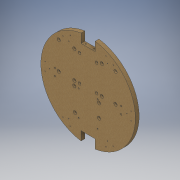
# Autodesk Inventor part: Platte3_neu
Saved by Autodesk Inventor 2017 SP1 (Build 210196100, 196)
## iProperties
Part Number: Platte3_neu
Material: Generisch
Document SubType Name: Modeling
Designer: Alex
Density: 1 g/cm^3
Appearance: Holzplatte
Author: Alex
Autodesk Inventor part; units mm, degrees
ref_plane "YZ Plane" through (0, 0, 0) normal (1, 0, 0) x (0, 1, 0)
ref_plane "XZ Plane" through (0, 0, 0) normal (0, 1, 0) x (-1, 0, 0)
ref_plane "XY Plane" through (0, 0, 0) normal (0, 0, 1) x (1, 0, 0)
sketch "Skizze1" plane through (0, 0, 0) normal (0, 1, 0) x (-1, 0, 0)
  circle A0 centre (0, 0) radius 100
  dimension "d0" = 200
  constraints: 1 centre point, 1 coincident
  measures "d0" diameter of A0
extrude "Extrusion1" add sketch "Skizze1" along normal blind 8
sketch "Skizze3" plane through (0, 0, 0) normal (0, -1, 0) x (1, 0, 0)
  point P0 (0, 0)
  point P1 (91, 8.85)
  point P2 (91, -8.85)
  point P3 (82, 0)
  point P4 (37.8357, 83.2333)
  point P5 (41, 71.0141)
  point P6 (53.1643, 74.3833)
  point P7 (-53.1643, 74.3833)
  point P8 (-41, 71.0141)
  point P9 (-37.8357, 83.2333)
  point P10 (-91, -8.85)
  point P11 (-82, 0)
  point P12 (-91, 8.85)
  point P13 (-37.8357, -83.2333)
  point P14 (-41, -71.0141)
  point P15 (-53.1643, -74.3833)
  point P16 (53.1643, -74.3833)
  point P17 (41, -71.0141)
  point P18 (37.8357, -83.2333)
  dimension "d3" = 17.7
  dimension "d4" = 9
  dimension "d5" = 8.85
  dimension "d6" = 82
  dimension "d9" = 360
  constraints: 1 horizontal alignment, 1 vertical alignment, 19 other
  measures "d3" distance of point (91, -8.85) point (91, 8.85)
  measures "d4" horizontal distance of point (82, 0) point (91, 8.85)
  measures "d5" vertical distance of point (82, 0) point (91, 8.85)
  measures "d6" distance of point (0, 0) point (82, 0)
hole "Bohrung1" at (91, 0, 8.85) at (91, 0, -8.85) at (82, 0, 0) at (37.8357, 0, 83.2333) at (41, 0, 71.0141) at (53.1643, 0, 74.3833) at (-53.1643, 0, 74.3833) at (-41, 0, 71.0141) at (-37.8357, 0, 83.2333) at (-91, 0, -8.85) at (-82, 0, 0) at (-91, 0, 8.85) at (-37.8357, 0, -83.2333) at (-41, 0, -71.0141) at (-53.1643, 0, -74.3833) at (53.1643, 0, -74.3833) at (41, 0, -71.0141) at (37.8357, 0, -83.2333) direction (0, 1, 0) diameter 1.5 depth 5 tip angle 118
sketch "Skizze4" plane through (0, 0, 0) normal (0, -1, 0) x (1, 0, 0)
  line L0 (0, 140.1034) -> (0, 25.1034)
  line L1 (0, 80) -> (15, 80)
  line L2 (15, 80) -> (15, 98.8686)
  circle A0 centre (0, 0) radius 100 projected
  arc A1 (15, 98.8686) -> (0, 100) centre (0, 0) ccw
  line L3 (0, 80) -> (-15, 80)
  line L4 (-15, 80) -> (-15, 98.8686)
  arc A2 (0, 100) -> (-15, 98.8686) centre (0, 0) ccw
  line L5 (0, -80) -> (-15, -80)
  line L6 (-15, -80) -> (-15, -98.8686)
  line L7 (0, -80) -> (15, -80)
  line L8 (15, -80) -> (15, -98.8686)
  arc A3 (-15, -98.8686) -> (0, -100) centre (0, 0) ccw
  arc A4 (0, -100) -> (15, -98.8686) centre (0, 0) ccw
  dimension "d18" = 15
  dimension "d20" = 80
  dimension "d27" = 15
  dimension "d28" = 15
  constraints: 18 end point, 8 point on circle, 4 centre point, 3 symmetric about line, 2 point on line, 1 coincident, 1 horizontal, 1 perpendicular, 1 vertical, 1 vertical alignment, 3 other
  measures "d18" distance of L1.start L1.end
  measures "d20" distance from line of point (0, 0) L1
  measures "d27" distance of L5.start L7.end
  measures "d28" distance of L5.start L5.end
extrude "Extrusion2" cut sketch "Skizze4" against normal blind 8 contours A0 L2 L1 L0 | L0 L3 L4 A0 | L6 L5 L7 L8 A0
sketch "Skizze5" plane through (-15, 0, 80) normal (0, 0, 1) x (1, 0, 0)
  line L0 (30, 8) -> (30, 0) projected
  line L1 (0, 8) -> (30, 8) projected
  point P0 (15, 0)
  point P1 (23.75, 4)
  point P2 (6.25, 4)
  dimension "d29" = 17.5
  dimension "d30" = 6.25
  dimension "d31" = 4
  constraints: 1 horizontal alignment
  measures "d29" distance of point (6.25, 4) point (23.75, 4)
  measures "d30" distance from line of point (23.75, 4) L0
  measures "d31" distance from line of L1 point (23.75, 4)
sketch "Skizze6" plane through (15, 0, -80) normal (0, 0, -1) x (-1, 0, 0)
  point P0 (15, 0)
  point P1 (6.25, 4)
  point P2 (23.75, 4)
hole "Bohrung2" at (8.75, 4, -80) at (-8.75, 4, -80) direction (0, 0, 1) diameter 2 depth 10 tip angle 118
hole "Bohrung3" at (8.75, 4, 80) at (-8.75, 4, 80) direction (0, 0, -1) diameter 2 depth 10 tip angle 118
sketch "Skizze11" plane through (0, 0, 0) normal (0, -1, 0) x (1, 0, 0)
  point P0 (0, 0)
  point P1 (20, -5)
  point P2 (-20, -5)
  point P3 (20, -59)
  point P4 (-20, -59)
  dimension "d81" = 40
  dimension "d82" = 20
  dimension "d83" = 5
  dimension "d84" = 54
  constraints: 2 horizontal alignment, 2 vertical alignment
  measures "d81" distance of point (-20, -5) point (20, -5)
  measures "d82" horizontal distance of point (0, 0) point (-20, -5)
  measures "d83" vertical distance of point (0, 0) point (-20, -5)
  measures "d84" distance of point (-20, -59) point (-20, -5)
hole "Bohrung5" at (20, 0, -5) at (-20, 0, -5) at (20, 0, -59) at (-20, 0, -59) direction (0, 1, 0) diameter 2.5 depth 8 tip angle 118
chamfer "Fase1" distance 2 angle 45 4 edges at (20, 8, -3.75) (-20, 8, -3.75) (-20, 8, -57.75) (20, 8, -57.75)
sketch "Skizze13" plane through (0, 0, 0) normal (0, -1, 0) x (1, 0, 0)
  point P0 (0, 0)
  point P1 (70, -7.5)
  point P2 (70, 7.5)
  point P3 (-70, -7.5)
  point P4 (-70, 7.5)
  dimension "d95" = 15
  dimension "d96" = 7.5
  dimension "d97" = 70
  dimension "d100" = 360
  constraints: 1 vertical alignment, 5 other
  measures "d95" distance of point (70, 7.5) point (70, -7.5)
  measures "d96" vertical distance of point (0, 0) point (70, -7.5)
  measures "d97" horizontal distance of point (0, 0) point (70, -7.5)
hole "Bohrung6" at (70, 0, -7.5) at (70, 0, 7.5) at (-70, 0, -7.5) at (-70, 0, 7.5) direction (0, 1, 0) diameter 3 depth 8 tip angle 118
chamfer "Fase2" distance 2 angle 45 4 edges at (70, 8, 9) (70, 8, -6) (-70, 8, -6) (-70, 8, 9)
sketch "Skizze14" plane through (0, 0, 0) normal (0, -1, 0) x (1, 0, 0)
  point P0 (0, 0)
  point P1 (29, -54)
  point P2 (29, -5)
  point P3 (-29, -5)
  point P4 (-29, -54)
  dimension "d112" = 49
  dimension "d113" = 58
  dimension "d114" = 5
  dimension "d115" = 29
  constraints: 2 horizontal alignment, 2 vertical alignment
  measures "d112" distance of point (-29, -5) point (-29, -54)
  measures "d113" distance of point (-29, -54) point (29, -54)
  measures "d114" vertical distance of point (0, 0) point (-29, -5)
  measures "d115" horizontal distance of point (0, 0) point (-29, -5)
hole "Bohrung7" [suppressed]
chamfer "Fase3" [suppressed]
sketch "Skizze15" plane through (0, 0, 0) normal (0, -1, 0) x (1, 0, 0)
  point P0 (0, 0)
  point P1 (58, 5)
  point P2 (58, 65)
  point P3 (29, 65)
  point P4 (29, 5)
  dimension "d126" = 29
  dimension "d127" = 60
  dimension "d128" = 5
  dimension "d129" = 29
  constraints: 2 horizontal alignment, 2 vertical alignment
  measures "d126" distance of point (29, 5) point (58, 5)
  measures "d127" distance of point (29, 65) point (29, 5)
  measures "d128" vertical distance of point (0, 0) point (29, 5)
  measures "d129" horizontal distance of point (0, 0) point (29, 5)
hole "Bohrung8" at (58, 0, 5) at (58, 0, 65) at (29, 0, 65) at (29, 0, 5) direction (0, 1, 0) diameter 3 depth 8 tip angle 118
chamfer "Fase4" distance 2 angle 45 4 edges at (29, 0, 6.5) (58, 0, 6.5) (58, 0, 66.5) (29, 0, 66.5)
sketch "Skizze16" plane through (0, 0, 0) normal (0, -1, 0) x (1, 0, 0)
  point P0 (0, 0)
  point P1 (-29, 5)
  point P2 (-29, 63)
  point P3 (-62, 63)
  point P4 (-62, 5)
  dimension "d140" = 33
  dimension "d141" = 58
  dimension "d142" = 5
  dimension "d143" = 29
  constraints: 2 horizontal alignment, 2 vertical alignment
  measures "d140" distance of point (-62, 5) point (-29, 5)
  measures "d141" distance of point (-29, 63) point (-29, 5)
  measures "d142" vertical distance of point (0, 0) point (-29, 5)
  measures "d143" horizontal distance of point (0, 0) point (-29, 5)
hole "Bohrung9" at (-29, 0, 5) at (-29, 0, 63) at (-62, 0, 63) at (-62, 0, 5) direction (0, 1, 0) diameter 3 depth 8 tip angle 118
chamfer "Fase5" distance 2 angle 45 4 edges at (-62, 0, 6.5) (-29, 0, 6.5) (-29, 0, 64.5) (-62, 0, 64.5)
sketch "Skizze17" plane through (0, 0, 0) normal (0, -1, 0) x (1, 0, 0)
  point P0 (0, 0)
  point P1 (-18, 5)
  point P2 (18, 5)
  point P3 (18, 61)
  point P4 (-18, 61)
  dimension "d154" = 56
  dimension "d155" = 36
  dimension "d156" = 18
  dimension "d157" = 5
  constraints: 2 horizontal alignment, 2 vertical alignment
  measures "d154" distance of point (-18, 61) point (-18, 5)
  measures "d155" distance of point (-18, 5) point (18, 5)
  measures "d156" horizontal distance of point (0, 0) point (-18, 5)
  measures "d157" vertical distance of point (0, 0) point (-18, 5)
hole "Bohrung10" at (-18, 0, 5) at (18, 0, 5) at (18, 0, 61) at (-18, 0, 61) direction (0, 1, 0) diameter 2 depth 8 tip angle 118
chamfer "Fase6" distance 2 angle 45 4 edges at (-18, 0, 6) (-18, 0, 62) (18, 0, 62) (18, 0, 6)
sketch "Skizze19" plane through (0, 0, 0) normal (0, -1, 0) x (1, 0, 0)
  circle A0 centre (-29, -5) radius 1.5 projected
  point P0 (0, 0)
  point P1 (-27.73, -53.277)
  point P2 (23.07, -38.02)
  point P3 (23.07, -10.08)
  dimension "d168" = 48.277
  dimension "d170" = 27.94
  dimension "d172" = 5.08
  dimension "d186" = 1.27
  dimension "d187" = 52.07
  constraints: 1 coincident, 1 vertical alignment
  measures "d168" vertical distance of point (-29, -5) point (-27.73, -53.277)
  measures "d170" distance of point (23.07, -10.08) point (23.07, -38.02)
  measures "d172" vertical distance of point (23.07, -10.08) point (-29, -5)
  measures "d186" horizontal distance of point (-27.73, -53.277) point (-29, -5)
  measures "d187" horizontal distance of point (-29, -5) point (23.07, -10.08)
hole "Bohrung11" at (-29, 0, -5) at (-27.73, 0, -53.277) at (23.07, 0, -38.02) at (23.07, 0, -10.08) direction (0, 1, 0) diameter 3 depth 8 tip angle 118
chamfer "Fase8" distance 2 angle 45 4 edges at (-27.73, 0, -51.777) (-29, 0, -3.5) (23.07, 0, -8.58) (23.07, 0, -36.52)
